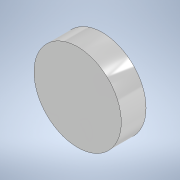
# Autodesk Inventor part: Bolt Cover
Saved by Autodesk Inventor 2021 (Build 250183000, 183)
## iProperties
Created: 2021-03-28
Part Number: Bolt Cover
Material: Aluminum 6061
Document SubType Name: Modeling
Designer: lucia
Density: 2.7 g/cm^3
Appearance: Aluminum - Polished
Author: lucia
Autodesk Inventor part; units mm, degrees
ref_plane "YZ Plane" through (0, 0, 0) normal (1, 0, 0) x (0, 1, 0)
ref_plane "XZ Plane" through (0, 0, 0) normal (0, 1, 0) x (-1, 0, 0)
ref_plane "XY Plane" through (0, 0, 0) normal (0, 0, 1) x (1, 0, 0)
sketch "Sketch3" plane through (0, 0, 0) normal (0, 0, 1) x (1, 0, 0)
  circle A0 centre (0, 0) radius 5.588
  dimension "d26" = 11.176
  constraints: 1 centre point, 1 coincident
  measures "d26" diameter of A0
extrude "Extrusion2" add sketch "Sketch3" along normal blind 3.175
equation "\"d9\" = 3.175"
body "Solid2"
